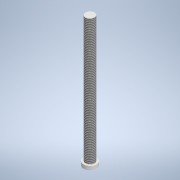
# Autodesk Inventor part: Tornillo_Corto
Saved by Autodesk Inventor 2021 (Build 250183000, 183)
## iProperties
Created: 2021-04-03
Part Number: Tornillo_Corto
Material: Genérico
Document SubType Name: Modeling
Designer: diego
Density: 1 g/cm^3
Appearance: Valor por defecto
Author: diego
Autodesk Inventor part; units mm, degrees
ref_plane "YZ Plane" through (0, 0, 0) normal (1, 0, 0) x (0, 1, 0)
ref_plane "XZ Plane" through (0, 0, 0) normal (0, 1, 0) x (-1, 0, 0)
ref_plane "XY Plane" through (0, 0, 0) normal (0, 0, 1) x (1, 0, 0)
sketch "Boceto1" plane through (0, 0, 0) normal (0, 1, 0) x (-1, 0, 0)
  circle A0 centre (0, 0) radius 3.5
  constraints: 1 centre point, 1 coincident
extrude "Extrusión1" add sketch "Boceto1" against normal blind 2
sketch "Boceto2" plane through (0, 0, 0) normal (0, 1, 0) x (1, 0, 0)
  circle A0 centre (0, 0) radius 2.45
  constraints: 1 centre point, 1 coincident
extrude "Extrusión2" add sketch "Boceto2" along normal blind 70
thread "Rosca1" size "M5x0.8" class "6g" standard "ANSI Metric M Profile" length 70
sketch "Boceto3" plane through (0, 70, 0) normal (0, 1, 0) x (1, 0, 0)
  circle A0 centre (0, 0) radius 2.5
  dimension "d8" = 5
  constraints: 1 centre point, 1 coincident
  measures "d8" diameter of A0
extrude "Extrusión3" cut sketch "Boceto3" against normal blind 25
sketch "Boceto4" plane through (0, 45, 0) normal (0, 1, 0) x (1, 0, 0)
  circle A0 centre (0, 0) radius 2.45
  constraints: 1 centre point, 1 coincident
extrude "Extrusión4" add sketch "Boceto4" along normal blind 12
sketch "Boceto5" plane through (0, 57, 0) normal (0, 1, 0) x (1, 0, 0)
  circle A0 centre (0, 0) radius 2.45
  constraints: 1 centre point, 1 coincident
extrude "Extrusión5" add sketch "Boceto5" along normal blind 12
sketch "Boceto6" plane through (0, 69, 0) normal (0, 1, 0) x (1, 0, 0)
  circle A0 centre (0, 0) radius 2.45
  constraints: 1 centre point, 1 coincident
extrude "Extrusión6" cut sketch "Boceto6" against normal blind 23
